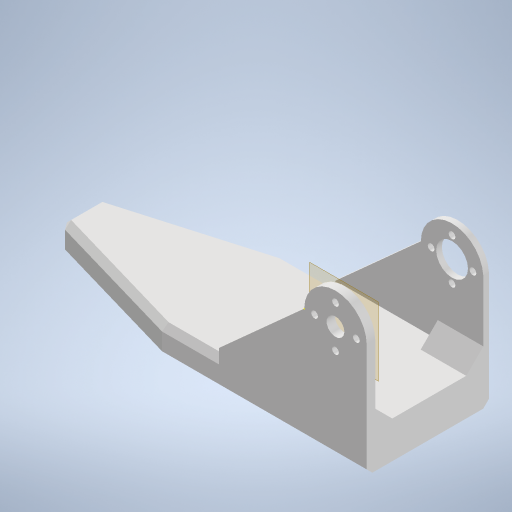
# Autodesk Inventor part: tibia
Saved by Autodesk Inventor 2024 (Build 280153000, 153)
## iProperties
Created: 2024-03-17
Part Number: tibia
Material: Genérico
Document SubType Name: Modeling
Designer: na_re
Density: 1 g/cm^3
Appearance: Valor por defecto
Author: na_re
Autodesk Inventor part; units mm, degrees
ref_plane "YZ Plane" through (0, 0, 0) normal (1, 0, 0) x (0, 1, 0)
ref_plane "XZ Plane" through (0, 0, 0) normal (0, 1, 0) x (-1, 0, 0)
ref_plane "XY Plane" through (0, 0, 0) normal (0, 0, 1) x (1, 0, 0)
ref_plane "Plano de trabajo1" through (0, 0, 0) normal (0, 0, 1) x (1, 0, 0)
sketch "Boceto1" plane through (0, 0, 0) normal (0, 0, 1) x (1, 0, 0)
  circle A0 centre (10.9923, 0) radius 10.9823 projected
  circle A1 centre (10.9923, 0) radius 3.1378 projected
  circle A2 centre (18.3423, 0) radius 1.2028 projected
  circle A3 centre (10.9923, 7.35) radius 1.2028 projected
  circle A4 centre (3.6423, 0) radius 1.2028 projected
  circle A5 centre (10.9923, -7.35) radius 1.2028 projected
  line L0 (0, 0) -> (0, 30)
  line L1 (21.9746, 0) -> (21.9746, -30)
  line L2 (0, 0) -> (0, -30)
  line L3 (0, -30) -> (21.9746, -30)
  circle A6 centre (10.9923, 0) radius 3.1378
  circle A7 centre (18.3423, 0) radius 1.2028
  circle A8 centre (10.9923, -7.35) radius 1.2028
  circle A9 centre (3.6423, 0) radius 1.2028
  circle A10 centre (10.9923, 7.35) radius 1.2028
  circle A11 centre (10.9923, 0) radius 10.9823
  line L4 (0, 0) -> (0, -30)
  line L5 (0, -30) -> (21.9746, -30)
  line L6 (21.9746, -30) -> (21.9746, 0)
  dimension "d0" = 30
  dimension "d1" = 30
  constraints: 14 end point, 6 centre point, 6 coincident, 5 concentric, 4 vertical, 2 perpendicular, 1 collinear, 1 horizontal, 1 horizontal alignment, 1 point on line, 1 tangent, 2 other
  measures "d0" distance of L0.start L0.end
  measures "d1" distance of L1.start L1.end
extrude "Extrusión1" add sketch "Boceto1" along normal blind 3
sketch "Boceto2" plane through (10.9923, 0, 3) normal (0, 0, 1) x (1, 0, 0)
  circle A0 centre (0, 0) radius 10.9823 projected
  line L0 (10.9823, 0) -> (10.9823, -30)
  line L1 (10.9823, -30) -> (-9.7118, -30)
  line L2 (-9.7118, -30) -> (-10.9923, 0)
  circle A1 centre (0, 0) radius 10.9823 projected
  circle A2 centre (0, -7.35) radius 1.2028 projected
  circle A3 centre (-7.35, 0) radius 1.2028 projected
  circle A4 centre (0, 7.35) radius 1.2028 projected
  circle A5 centre (7.35, 0) radius 1.2028 projected
  circle A6 centre (0, 0) radius 3.1378 projected
  point P0 (-10.9723, -0.4683)
  dimension "d4" = 30
  constraints: 6 end point, 2 vertical, 1 perpendicular, 3 other
  measures "d4" distance of L0.start L0.end
extrude "Extrusión2" add sketch "Boceto2" against normal blind 3 contours L0 L1 L2 A0
sketch "Boceto3" plane through (0, 0, 0) normal (0, 0, -1) x (-1, 0, 0)
  point P0 (0, 0)
sketch "Boceto4" plane through (0, 0, 3) normal (0, 0, 1) x (1, 0, 0)
  point P0 (0, 0)
sketch "Boceto5" plane through (0, 0, 0) normal (0, 0, -1) x (-1, 0, 0)
  arc A0 (-0.02, -0.4683) -> (-21.9746, 0) centre (-10.9923, 0) ccw projected
  line L0 (-21.9746, 0) -> (-21.9746, -30) projected
  line L1 (-21.9746, -30) -> (-1.2805, -30) projected
  line L2 (-1.2805, -30) -> (-0.02, -0.4683) projected
  circle A1 centre (-10.9923, -7.35) radius 1.2028 projected
  circle A2 centre (-3.6423, 0) radius 1.2028 projected
  circle A3 centre (-10.9923, 7.35) radius 1.2028 projected
  circle A4 centre (-18.3423, 0) radius 1.2028 projected
  circle A5 centre (-10.9923, 0) radius 3.1378 projected
  line L3 (-21.9746, -30) -> (0, -30)
  line L4 (0, -30) -> (0, 0)
  line L5 (0, 0) -> (-21.9746, 0)
  line L6 (-21.9746, 0) -> (-21.9746, -30)
  point P0 (-0.01, 0)
  constraints: 8 end point, 2 parallel, 1 horizontal, 1 perpendicular
extrude "Extrusión3" add sketch "Boceto5" against normal blind 3 contours A0 L5 L4 L3 L2
sketch "Boceto6" plane through (0, 0, 0) normal (0, 0, -1) x (-1, 0, 0)
  point P0 (0, 0)
sketch "Boceto7" plane through (0, 0, 0) normal (0, 0, -1) x (-1, 0, 0)
  line L0 (-21.9746, -30) -> (0, -30) projected
  line L1 (-21.9746, -30) -> (-21.9746, 0) projected
  line L2 (0, -30) -> (-21.9746, -30)
  line L3 (-21.9746, -30) -> (-21.9746, -27)
  line L4 (-21.9746, -27) -> (0, -27)
  line L5 (0, -27) -> (0, -30)
  point P0 (0, 0)
  dimension "d9" = 3
  constraints: 8 end point, 2 parallel, 1 horizontal, 1 perpendicular, 1 point on line
  measures "d9" distance of L2.end L3.end
extrude "Extrusión4" add sketch "Boceto7" along normal blind 40
sketch "Boceto8" plane through (0, -27, 0) normal (0, 1, 0) x (1, 0, 0)
  line L0 (0, -3) -> (0, 40) projected
  line L1 (21.9746, -3) -> (21.9746, 40) projected
  line L2 (0, 40) -> (21.9746, 40)
  line L3 (21.9746, 40) -> (21.9746, 38)
  line L4 (21.9746, 38) -> (0, 38)
  line L5 (0, 38) -> (0, 40)
  point P0 (0, 0)
  point P1 (21.9746, 40)
  point P2 (0, 38)
  dimension "d12" = 2
  constraints: 8 end point, 2 parallel, 1 horizontal, 1 perpendicular, 1 point on line
  measures "d12" distance of L2.end L3.end
extrude "Extrusión5" add sketch "Boceto8" along normal blind 40
sketch "Boceto9" plane through (0, 0, -40) normal (0, 0, -1) x (-1, 0, 0)
  circle A0 centre (-11.0072, -0.015) radius 2.7 projected
  circle A1 centre (-11.0099, -0.0117) radius 10.9823 projected
  circle A2 centre (-18.3423, 0) radius 1.2028 projected
  circle A3 centre (-10.9923, -7.35) radius 1.2028 projected
  circle A4 centre (-10.9923, 7.35) radius 1.2028 projected
  circle A5 centre (-3.6423, 0) radius 1.2028 projected
  line L0 (-21.9746, -30) -> (-21.9746, 13) projected
  line L1 (-21.9746, -30) -> (0, -30) projected
  line L2 (0, -30) -> (0, 13) projected
  line L3 (-21.9746, 13) -> (0, 13) projected
  line L4 (-21.5706, 0) -> (-25.972, 0)
  line L5 (-25.972, 0) -> (-25.972, 18.1609)
  line L6 (-25.972, 18.1609) -> (4.5124, 18.1609)
  line L7 (4.5124, 18.1609) -> (4.5124, 1.2028)
  line L8 (4.5124, 1.2028) -> (4.5124, 0)
  line L9 (-3.6423, 0) -> (4.822, 0)
  point P0 (0, 0)
  point P1 (-21.9746, 0.6093)
  point P2 (-0.0276, 0)
  point P3 (0, 0)
  constraints: 12 end point, 3 perpendicular, 3 point on line, 1 horizontal
extrude "Extrusión6" cut sketch "Boceto9" against normal blind 40 contours A0 | A1 L0 L3 L2 L9 | A2 | A3 | A4 | A5
sketch "Boceto10" plane through (0, -30, 3) normal (0, -1, 0) x (1, 0, 0)
  point P0 (0, -3)
sketch "Boceto11" plane through (0, -30, 3) normal (0, -1, 0) x (1, 0, 0)
  line L0 (0.0276, -43) -> (21.9746, -43) projected
  line L1 (0, -3) -> (0, 0) projected
  line L2 (21.9746, -43) -> (0, -43)
  line L3 (0, -43) -> (0, 0)
  line L4 (0, 0) -> (21.9746, 0)
  line L5 (21.9746, 0) -> (21.9746, -43)
  line L6 (0, -43) -> (-100, -43)
  line L7 (-100, -43) -> (-100, 0)
  line L8 (-100, 0) -> (0, 0)
  line L9 (0, 0) -> (0, -43)
  line L10 (-100, 0) -> (-100, -21.5)
  line L11 (-100, -21.5) -> (-100, -14.5)
  line L12 (-100, -14.5) -> (-100, -28.5)
  line L13 (-100, -28.5) -> (-50, -43)
  line L14 (-50, -43) -> (-50, 0)
  line L15 (-100, -14.5) -> (-50, 0)
  dimension "d17" = 100
  dimension "d18" = 21.5
  dimension "d19" = 7
  dimension "d20" = 14
  constraints: 28 end point, 4 parallel, 3 midpoint, 3 point on line, 2 horizontal, 2 perpendicular
  measures "d17" distance of L7.end L8.end
  measures "d18" distance of L7.end L10.end
  measures "d19" distance of L10.end L11.end
  measures "d20" distance of L11.end L12.end
extrude "Extrusión7" add sketch "Boceto11" along normal blind 10 contours L2 L3 L1 L4 L5 L0 | L6 L14 L8 L1 L3 | L13 L7 L15 L14
chamfer "Chaflán1" distance 2 angle 45 12 edges at (-14.0127, -40, -40) (-75, -40, -32.75) (-75, -30, -32.75) (-25, -30, -40) (-14.0127, -40, 3) (-75, -40, -4.25) (-100, -40, -18.5) (-75, -30, -4.25) (-25, -30, 3) (-100, -30, -18.5) (-100, -35, -25.5) (-100, -35, -11.5)
sketch "Boceto12" plane through (0, -40, 3) normal (0, -1, 0) x (1, 0, 0)
  line L0 (-49.7159, -2) -> (21.9746, -2) projected
  line L1 (-98, -16.0024) -> (-49.7159, -2) projected
  line L2 (-98, -26.9976) -> (-98, -16.0024) projected
  line L3 (-49.7159, -41) -> (-98, -26.9976) projected
  line L4 (21.9746, -41) -> (-49.7159, -41) projected
  line L5 (21.9746, -41) -> (21.9746, -2) projected
  line L6 (-48.5793, -33) -> (-88.2344, -21.5)
  line L7 (-88.2344, -21.5) -> (-48.5793, -10)
  line L8 (-48.5793, -10) -> (13.9746, -10)
  line L9 (13.9746, -10) -> (13.9746, -33)
  line L10 (13.9746, -33) -> (-48.5793, -33)
  point P0 (0, -3)
  dimension "d26" = 8
  constraints: 10 end point, 4 other
  measures "d26" distance between parallel lines of L4 L10
extrude "Extrusión8" cut sketch "Boceto12" against normal blind 4 contours L6 L7 L8 L9 L10
sketch "Boceto13" plane through (0, 0, -40) normal (0, 0, -1) x (-1, 0, 0)
  circle A0 centre (-11.0099, -0.0117) radius 5.6 projected
  circle A1 centre (-11.0072, -0.015) radius 2.7 projected
  point P0 (0, 0)
extrude "Extrusión9" cut sketch "Boceto13" against normal blind 5
sketch "Boceto14" plane through (0, 0, 0) normal (-1, 0, 0) x (0, 0, 1)
  line L0 (0, -27) -> (-38, -27) projected
  line L1 (-38, 0) -> (-40, 0) projected
  line L2 (-40, -32) -> (-40, 0) projected
  line L3 (-38, -30) -> (-40, -32) projected
  line L4 (1, -30) -> (-38, -30) projected
  line L5 (3, -32) -> (1, -30) projected
  line L6 (3, 0) -> (3, -32) projected
  line L7 (0, 0) -> (3, 0) projected
  line L8 (0, -27) -> (0, 0) projected
  line L9 (0, -27) -> (-38, -27) projected
  line L10 (-38, -27) -> (-38, 0) projected
  point P0 (0, 0)
extrude "Extrusión10" add sketch "Boceto14" along normal blind 30
sketch "Boceto15" plane through (0, 0, 3) normal (0, 0, 1) x (1, 0, 0)
  line L0 (21.9746, -38) -> (-50, -38) projected
  line L1 (21.9746, -38) -> (21.9746, 0) projected
  arc A0 (21.9746, 0) -> (0.01, 0) centre (10.9923, 0) ccw projected
  line L2 (0.01, 0) -> (-30, 0) projected
  line L3 (-30, -32) -> (-30, 0) projected
  line L4 (-50, -32) -> (-30, -32) projected
  line L5 (-50, -32) -> (-50, -38) projected
  circle A1 centre (10.9923, -7.35) radius 1.2028 projected
  circle A2 centre (3.6423, 0) radius 1.2028 projected
  circle A3 centre (10.9923, 7.35) radius 1.2028 projected
  circle A4 centre (18.3423, 0) radius 1.2028 projected
  circle A5 centre (10.9923, 0) radius 3.1378 projected
  line L6 (21.9746, -27) -> (-30, -27) projected
  line L7 (0.01, 0) -> (-30, -27)
  point P0 (0, 0)
  constraints: 2 end point
extrude "Extrusión11" cut sketch "Boceto15" against normal blind 100 contours L3 L2 L7
chamfer "Chaflán2" distance 2 angle 45 1 edges at (-30, -27, -19)
sketch "Boceto16" plane through (21.9746, -27, 0) normal (0, 1, 0) x (1, 0, 0)
  line L0 (-49.9746, 0) -> (-49.9746, 38) projected
  line L1 (0, 0) -> (-49.9746, 0) projected
  line L2 (0, 0) -> (0, 38) projected
  line L3 (0, 38) -> (-49.9746, 38) projected
  line L4 (0, 0) -> (-16, 0)
  line L5 (-16, 0) -> (-16, 6)
  line L6 (-16, 6) -> (0, 6)
  line L7 (0, 6) -> (0, 0)
  line L8 (0, 38) -> (-16, 38)
  line L9 (-16, 38) -> (-16, 32)
  line L10 (-16, 32) -> (0, 32)
  line L11 (0, 32) -> (0, 38)
  point P0 (-21.9746, 0)
  dimension "d38" = 16
  dimension "d39" = 6
  dimension "d40" = 16
  dimension "d41" = 6
  constraints: 16 end point, 4 parallel, 2 horizontal, 2 perpendicular
  measures "d38" distance of L5.end L6.end
  measures "d39" distance of L4.end L5.end
  measures "d40" distance of L10.end L9.end
  measures "d41" distance of L9.end L8.end
extrude "Extrusión12" add sketch "Boceto16" along normal blind 6 contours L5 L6 L2 L1 | L3 L2 L10 L9
chamfer "Chaflán3" distance 6 angle 45 2 edges at (13.9746, -21, -6) (13.9746, -21, -32)
